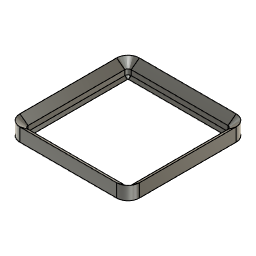
GridfinityBase v1 (Autodesk Fusion 360 design; units mm, degrees)
Autodesk Fusion 360 part; units mm, degrees
sketch "Sketch1" plane through (0, 0, 0) normal (0, 0, 1) x (1, 0, 0)
  line L0 (17, 21) -> (-17, 21)
  line L1 (-21, 17) -> (-21, -17)
  line L2 (-17, -21) -> (17, -21)
  line L3 (21, -17) -> (21, 17)
  line L4 (21, 21) -> (-21, -21) construction
  line L5 (-21, 21) -> (21, -21) construction
  arc A0 (-17, 21) -> (-21, 17) centre (-17, 17) ccw
  arc A1 (21, 17) -> (17, 21) centre (17, 17) ccw
  arc A2 (17, -21) -> (21, -17) centre (17, -17) ccw
  arc A3 (-21, -17) -> (-17, -21) centre (-17, -17) ccw
  dimension "d1" = 42
  dimension "d2" = 42
  dimension "d11" = 4
  constraint horizontal L0
  constraint perpendicular L0 L1
  constraint parallel L0 L2
  constraint parallel L1 L3
  constraint coincident L4 origin
  constraint coincident L5 origin
  constraint coincident L5.start L1
  constraint coincident L5.start L0
  constraint tangent L1 A0
  constraint tangent L0 A0
  constraint coincident L4.start L0
  constraint coincident L4.start L3
  constraint tangent L0 A1
  constraint tangent L3 A1
  constraint equal A0 A1
  constraint coincident L5.end L3
  constraint coincident L5.end L2
  constraint tangent L3 A2
  constraint tangent L2 A2
  constraint equal A0 A2
  constraint coincident L4.end L2
  constraint coincident L4.end L1
  constraint tangent L2 A3
  constraint tangent L1 A3
  constraint equal A0 A3
  measures "d1" distance of L4.end L5.end
  measures "d2" distance of L5.start L4.end
  measures "d11" radius of A0
sketch "Sketch3" plane through (0, 0, 0) normal (1, 0, 0) x (0, 1, 0)
  line L0 (-20.9874, -0.0027) -> (-20.9874, 4.6473)
  line L1 (-20.9874, 4.6473) -> (-18.1302, 2.4973)
  line L2 (-18.1302, 2.4973) -> (-18.1302, 0.7)
  line L3 (-18.1302, 0.7) -> (-17.2, 0)
  line L4 (-17.2, 0) -> (-20.9874, -0.0027)
  dimension "d8" = 0.7
  dimension "d9" = 2.15
  dimension "d10" = 4.65
  constraint vertical L0
  constraint parallel L0 L2
  constraint parallel L1 L3
  measures "d8" vertical distance of L2.end L3.end
  measures "d9" vertical distance of L0.end L1.end
  measures "d10" distance of L0.start L0.end
sweep "Sweep1" add profiles "Sketch3" path "Sketch1" along L3 A1 L0 A0 L1 A3 L2 A2 section 1
